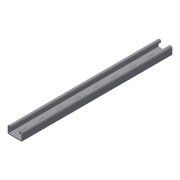
# Autodesk Inventor part: c channel for mounting plate 760 first hole
Saved by Autodesk Inventor 2015 (Build 190159000, 159)
## iProperties
Created: 2014-02-01
Part Number: c channel for mounting plate 760 first hole
Material: Generic
Document SubType Name: Modeling
Designer: Alex
Density: 1 g/cm^3
Appearance: Default
Author: Alex
Autodesk Inventor part; units mm, degrees
ref_plane "YZ Plane" through (0, 0, 0) normal (1, 0, 0) x (0, 1, 0)
ref_plane "XZ Plane" through (0, 0, 0) normal (0, 1, 0) x (-1, 0, 0)
ref_plane "XY Plane" through (0, 0, 0) normal (0, 0, 1) x (1, 0, 0)
ref_plane "Work Plane1" through (0, 0, 0) normal (0, 0, 1) x (1, 0, 0)
sketch "Sketch1" plane through (0, 0, 0) normal (0, 0, 1) x (1, 0, 0)
  arc A0 (-113.2188, 0) -> (-109.7581, 3.4607) centre (-113.2188, 3.4607) ccw projected
  line L0 (-109.7581, 17.1767) -> (-109.7581, 3.4607) projected
  arc A1 (-109.7581, 17.1767) -> (-114.8063, 22.225) centre (-114.8063, 17.1767) ccw projected
  line L1 (-115.8223, 22.225) -> (-114.8063, 22.225) projected
  arc A2 (-115.8223, 22.225) -> (-119.2831, 18.7642) centre (-115.8223, 18.7642) ccw projected
  line L2 (-119.2831, 16.4211) -> (-119.2831, 18.7642) projected
  arc A3 (-119.2831, 16.4211) -> (-116.6161, 16.4211) centre (-117.9496, 16.4211) ccw projected
  line L3 (-116.6161, 18.7642) -> (-116.6161, 16.4211) projected
  arc A4 (-115.8223, 19.558) -> (-116.6161, 18.7642) centre (-115.8223, 18.7642) ccw projected
  line L4 (-114.8063, 19.558) -> (-115.8223, 19.558) projected
  arc A5 (-112.4251, 17.1767) -> (-114.8063, 19.558) centre (-114.8063, 17.1767) ccw projected
  line L5 (-112.4251, 3.4607) -> (-112.4251, 17.1767) projected
  arc A6 (-113.2188, 2.667) -> (-112.4251, 3.4607) centre (-113.2188, 3.4607) ccw projected
  line L6 (-147.5723, 2.667) -> (-113.2188, 2.667) projected
  arc A7 (-148.3661, 3.4607) -> (-147.5723, 2.667) centre (-147.5723, 3.4607) ccw projected
  line L7 (-148.3661, 17.1767) -> (-148.3661, 3.4607) projected
  arc A8 (-145.9848, 19.558) -> (-148.3661, 17.1767) centre (-145.9848, 17.1767) ccw projected
  line L8 (-144.9688, 19.558) -> (-145.9848, 19.558) projected
  arc A9 (-144.1751, 18.7642) -> (-144.9688, 19.558) centre (-144.9688, 18.7642) ccw projected
  line L9 (-144.1751, 16.4211) -> (-144.1751, 18.7642) projected
  arc A10 (-144.1751, 16.4211) -> (-141.5081, 16.4211) centre (-142.8416, 16.4211) ccw projected
  line L10 (-141.5081, 18.7642) -> (-141.5081, 16.4211) projected
  arc A11 (-141.5081, 18.7642) -> (-144.9688, 22.225) centre (-144.9688, 18.7642) ccw projected
  line L11 (-145.9848, 22.225) -> (-144.9688, 22.225) projected
  arc A12 (-145.9848, 22.225) -> (-151.0331, 17.1767) centre (-145.9848, 17.1767) ccw projected
  line L12 (-151.0331, 3.4607) -> (-151.0331, 17.1767) projected
  arc A13 (-151.0331, 3.4607) -> (-147.5723, 0) centre (-147.5723, 3.4607) ccw projected
  line L13 (-113.2188, 0) -> (-147.5723, 0) projected
  point P0 (0, 0)
extrude "Extrusion1" add sketch "Sketch1" along normal blind 417.9316
ref_plane "Work Plane2" through (0, 0, 208.9658) normal (0, 0, 1) x (1, 0, 0)
sketch "Sketch2" plane through (-147.5723, 0, 0) normal (0, -1, 0) x (1, 0, 0)
  line L0 (17.1768, 26.4541) -> (17.1768, 40.7289) construction
  line L1 (6.0642, 0) -> (6.0642, 417.9316) projected
  line L2 (10.0267, 26.4541) -> (10.0267, 40.7289)
  line L3 (24.3269, 40.7289) -> (24.3269, 26.4541)
  arc A0 (10.0267, 26.4541) -> (24.3269, 26.4541) centre (17.1768, 26.4541) ccw
  arc A1 (24.3269, 40.7289) -> (10.0267, 40.7289) centre (17.1768, 40.7289) ccw
  line L4 (0, 0) -> (34.3535, 0) construction
  line L5 (17.1768, 0) -> (17.1767, 417.9316) construction
  line L6 (34.3535, 417.9316) -> (0, 417.9316) construction
  line L7 (10.0267, 77.2541) -> (10.0267, 91.5289)
  line L8 (24.3269, 91.5289) -> (24.3269, 77.2541)
  arc A2 (10.0267, 77.2541) -> (24.3269, 77.2541) centre (17.1768, 77.2541) ccw
  arc A3 (24.3269, 91.5289) -> (10.0267, 91.5289) centre (17.1768, 91.5289) ccw
  line L9 (17.1768, 50.8) -> (17.1767, 468.7316) construction
  line L10 (10.0266, 128.0541) -> (10.0266, 142.3289)
  line L11 (24.3268, 142.3289) -> (24.3268, 128.0541)
  arc A4 (10.0266, 128.0541) -> (24.3268, 128.0541) centre (17.1767, 128.0541) ccw
  arc A5 (24.3268, 142.3289) -> (10.0266, 142.3289) centre (17.1767, 142.3289) ccw
  line L12 (17.1768, 101.6) -> (17.1767, 519.5316) construction
  line L13 (10.0266, 178.8541) -> (10.0266, 193.1289)
  line L14 (24.3268, 193.1289) -> (24.3268, 178.8541)
  arc A6 (10.0266, 178.8541) -> (24.3268, 178.8541) centre (17.1767, 178.8541) ccw
  arc A7 (24.3268, 193.1289) -> (10.0266, 193.1289) centre (17.1767, 193.1289) ccw
  line L15 (17.1767, 152.4) -> (17.1767, 570.3316) construction
  line L16 (10.0266, 229.6541) -> (10.0266, 243.9289)
  line L17 (24.3268, 243.9289) -> (24.3268, 229.6541)
  arc A8 (10.0266, 229.6541) -> (24.3268, 229.6541) centre (17.1767, 229.6541) ccw
  arc A9 (24.3268, 243.9289) -> (10.0266, 243.9289) centre (17.1767, 243.9289) ccw
  line L18 (17.1767, 203.2) -> (17.1767, 621.1316) construction
  line L19 (10.0266, 280.4541) -> (10.0266, 294.7289)
  line L20 (24.3268, 294.7289) -> (24.3268, 280.4541)
  arc A10 (10.0266, 280.4541) -> (24.3268, 280.4541) centre (17.1767, 280.4541) ccw
  arc A11 (24.3268, 294.7289) -> (10.0266, 294.7289) centre (17.1767, 294.7289) ccw
  line L21 (17.1767, 254) -> (17.1767, 671.9316) construction
  line L22 (10.0266, 331.2541) -> (10.0266, 345.5289)
  line L23 (24.3268, 345.5289) -> (24.3268, 331.2541)
  arc A12 (10.0266, 331.2541) -> (24.3268, 331.2541) centre (17.1767, 331.2541) ccw
  arc A13 (24.3268, 345.5289) -> (10.0266, 345.5289) centre (17.1767, 345.5289) ccw
  line L24 (17.1767, 304.8) -> (17.1767, 722.7316) construction
  line L25 (10.0266, 382.0541) -> (10.0266, 396.3289)
  line L26 (24.3268, 396.3289) -> (24.3268, 382.0541)
  arc A14 (10.0266, 382.0541) -> (24.3268, 382.0541) centre (17.1767, 382.0541) ccw
  arc A15 (24.3268, 396.3289) -> (10.0266, 396.3289) centre (17.1767, 396.3289) ccw
  line L27 (17.1767, 355.6) -> (17.1767, 773.5316) construction
  point P0 (147.5723, 0)
  point P1 (17.1768, 33.5915)
  point P2 (17.1768, 84.3915)
  point P3 (17.1768, 135.1915)
  point P4 (17.1767, 185.9915)
  point P5 (17.1767, 236.7915)
  point P6 (17.1767, 287.5915)
  point P7 (17.1767, 338.3915)
  point P8 (17.1767, 389.1915)
  dimension "d2" = 14.3002
  dimension "d3" = 14.2748
  dimension "d4" = 26.4541
  dimension "d7" = 50.8
  constraints: 52 end point, 32 point on circle, 16 centre point, 8 point on line, 4 tangent, 3 midpoint, 2 parallel, 1 collinear, 1 vertical, 97 other
  measures "d2" distance between parallel lines of L2 L3
  measures "d3" distance of L0.end L0.start
  measures "d4" distance of L0.start L5.start
  measures "d7" distance of L5.start L9.start
extrude "Extrusion2" cut sketch "Sketch2" against normal blind 25.4
body "Solid1"
